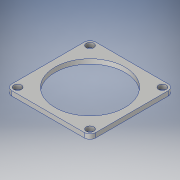
# Autodesk Inventor part: Bearing Block P2
Saved by Autodesk Inventor 2019.4 (Build 234330000, 330)
## iProperties
Created: 2019-12-12
Part Number: Bearing Block P2
Material: Aluminum 6061
Document SubType Name: Modeling
Designer: admin
Density: 2.7 g/cm^3
Appearance: Aluminum - Flat
Author: admin
Autodesk Inventor part; units mm, degrees
ref_plane "YZ Plane" through (0, 0, 0) normal (1, 0, 0) x (0, 1, 0)
ref_plane "XZ Plane" through (0, 0, 0) normal (0, 1, 0) x (-1, 0, 0)
ref_plane "XY Plane" through (0, 0, 0) normal (0, 0, 1) x (1, 0, 0)
sketch "Sketch1" plane through (0, 0, 0) normal (0, 1, 0) x (-1, 0, 0)
  line L0 (-18, 18) -> (18, 18)
  line L1 (18, 18) -> (18, -18)
  line L2 (18, -18) -> (-18, -18)
  line L3 (-18, -18) -> (-18, 18)
  line L4 (-18, 18) -> (18, -18) construction
  line L5 (18, 18) -> (-18, -18) construction
  circle A0 centre (15.5, -15.5) radius 1.65
  circle A1 centre (15.5, 15.5) radius 1.65
  circle A2 centre (-15.5, 15.5) radius 1.65
  circle A3 centre (-15.5, -15.5) radius 1.65
  circle A4 centre (0, 0) radius 15
  dimension "d0" = 36
  dimension "d1" = 36
  dimension "d2" = 3.3
  dimension "d3" = 3.3
  dimension "d4" = 3.3
  dimension "d5" = 3.3
  dimension "d6" = 2.5
  dimension "d7" = 2.5
  dimension "d8" = 2.5
  dimension "d9" = 2.5
  dimension "d10" = 30
  constraints: 12 end point, 5 centre point, 4 point on line, 2 midpoint, 2 parallel, 1 coincident, 1 horizontal, 1 perpendicular
  measures "d0" distance of L1.end L2.end
  measures "d1" distance of L0.end L1.end
  measures "d2" diameter of A0
  measures "d3" diameter of A1
  measures "d4" diameter of A2
  measures "d5" diameter of A3
  measures "d6" distance from line of L1 A0.centre
  measures "d7" distance from line of L0 A1.centre
  measures "d8" distance from line of L3 A2.centre
  measures "d9" distance from line of L2 A3.centre
  measures "d10" diameter of A4
extrude "Extrusion1" add sketch "Sketch1" along normal blind 2
fillet "Fillet1" radius 2.5 4 edges at (-18, 1, 18) (18, 1, 18) (18, 1, -18) (-18, 1, -18)
body "Solid1"
